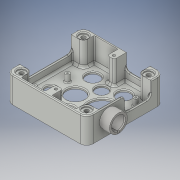
# Autodesk Inventor part: NUCBasePCB
Saved by Autodesk Inventor 2016 (Build 200138000, 138)
## iProperties
Created: 2015-09-23
Part Number: NUCBasePCB
Material: Generic
Document SubType Name: Modeling
Designer: lachesis
Density: 1 g/cm^3
Appearance: Default
Author: lachesis
Autodesk Inventor part; units mm, degrees
ref_plane "YZ Plane" through (0, 0, 0) normal (1, 0, 0) x (0, 1, 0)
ref_plane "XZ Plane" through (0, 0, 0) normal (0, 1, 0) x (-1, 0, 0)
ref_plane "XY Plane" through (0, 0, 0) normal (0, 0, 1) x (1, 0, 0)
sketch "Sketch1" plane through (0, 0, 0) normal (0, 1, 0) x (-1, 0, 0)
  line L0 (58.42, 56.134) -> (-58.42, 56.134)
  line L1 (-58.42, 56.134) -> (-58.42, -56.134)
  line L2 (-58.42, -56.134) -> (58.42, -56.134)
  line L3 (58.42, -56.134) -> (58.42, 56.134)
  point P0 (0, 0)
  point P1 (0, -56.134)
  point P2 (58.42, 0)
  dimension "d0" = 112.268
  dimension "d1" = 116.84
  constraints: 8 end point, 2 midpoint, 2 parallel, 1 horizontal, 1 horizontal alignment, 1 perpendicular, 1 vertical alignment
  measures "d0" distance of L2.end L0.start
  measures "d1" distance of L1.end L2.end
extrude "Extrusion1" add sketch "Sketch1" along normal blind 37.335
sketch "Sketch2" plane through (0, 37.335, 0) normal (0, 1, 0) x (1, 0, 0)
  line L0 (58.42, -56.134) -> (58.42, 56.134) projected
  line L1 (58.42, 56.134) -> (-58.42, 56.134) projected
  line L2 (-58.42, -56.134) -> (58.42, -56.134) projected
  line L3 (-58.42, 56.134) -> (-58.42, -56.134) projected
  point P0 (0, 0)
  point P1 (47.244, 44.958)
  point P2 (47.244, -44.958)
  point P3 (-47.244, 44.958)
  point P4 (-47.244, -44.958)
  dimension "d4" = 11.176
  dimension "d5" = 11.176
  dimension "d6" = 11.176
  dimension "d7" = 11.176
  constraints: 2 horizontal alignment, 2 vertical alignment
  measures "d4" distance from line of L0 point (47.244, 44.958)
  measures "d5" distance from line of L1 point (47.244, 44.958)
  measures "d6" distance from line of L2 point (-47.244, -44.958)
  measures "d7" distance from line of L3 point (-47.244, -44.958)
hole "Hole1" at (47.244, 37.335, -44.958) at (47.244, 37.335, 44.958) at (-47.244, 37.335, -44.958) at (-47.244, 37.335, 44.958) direction (0, -1, 0) diameter 3.302 end through all counterbore diameter 5.969 counterbore depth 31.75
sketch "Sketch3" plane through (0, 37.335, 0) normal (0, 1, 0) x (1, 0, 0)
  circle A0 centre (47.244, 44.958) radius 2.9845 projected
  circle A1 centre (47.244, -44.958) radius 2.9845 projected
  circle A2 centre (-47.244, 44.958) radius 2.9845 projected
  circle A3 centre (-47.244, -44.958) radius 2.9845 projected
  circle A4 centre (47.244, 44.958) radius 1.651 projected
  circle A5 centre (47.244, -44.958) radius 1.651 projected
  circle A6 centre (-47.244, -44.958) radius 1.651 projected
  point P0 (0, 0)
  constraints: 4 coincident
hole "Hole2" at (47.244, 37.335, -44.958) at (47.244, 37.335, 44.958) at (-47.244, 37.335, 44.958) at (-47.244, 37.335, -44.958) direction (0, -1, 0) diameter 12.065 depth 2.413
sketch "Sketch5" plane through (0, 0, 0) normal (0, -1, 0) x (1, 0, 0)
  circle A0 centre (-47.244, 44.958) radius 1.651 projected
  circle A1 centre (-47.244, -44.958) radius 1.651 projected
  point P0 (0, 0)
  point P1 (0, 42.164)
  point P2 (0, -42.164)
  dimension "d25" = 47.244
  dimension "d26" = 2.794
  dimension "d27" = 2.794
  constraints: 1 vertical alignment
  measures "d25" horizontal distance of A0.centre point (0, 42.164)
  measures "d26" vertical distance of A0.centre point (0, 42.164)
  measures "d27" vertical distance of A1.centre point (0, -42.164)
hole "Hole3" at (0, 0, 42.164) at (0, 0, -42.164) direction (0, 1, 0) diameter 3.9116 end through all counterbore diameter 6.604 counterbore depth 25.146
sketch "Sketch6" plane through (0, 37.335, 0) normal (0, 1, 0) x (1, 0, 0)
  circle A0 centre (0, -42.164) radius 1.9558 projected
  circle A1 centre (0, 42.164) radius 1.9558 projected
  circle A2 centre (-47.244, -44.958) radius 6.0325 projected
  circle A3 centre (47.244, 44.958) radius 6.0325 projected
  circle A4 centre (47.244, -44.958) radius 6.0325 projected
  circle A5 centre (-47.244, 44.958) radius 6.0325 projected
  line L0 (-58.42, -56.134) -> (58.42, -56.134) projected
  line L1 (58.42, -56.134) -> (58.42, 56.134) projected
  line L2 (58.42, 56.134) -> (-58.42, 56.134) projected
  line L3 (-58.42, 56.134) -> (-58.42, -56.134) projected
  line L4 (39.624, 52.959) -> (39.624, 37.338)
  line L5 (39.624, 37.338) -> (55.245, 37.338)
  line L6 (55.245, 37.338) -> (55.245, -37.338)
  line L7 (55.245, -37.338) -> (39.624, -37.338)
  line L8 (39.624, -37.338) -> (39.624, -52.959)
  line L9 (-39.624, -52.959) -> (-39.624, -37.338)
  line L10 (-39.624, -37.338) -> (-55.245, -37.338)
  line L11 (-55.245, -37.338) -> (-55.245, 37.338)
  line L12 (-55.245, 37.338) -> (-39.624, 37.338)
  line L13 (-39.624, 37.338) -> (-39.624, 52.959)
  line L14 (-39.624, -52.959) -> (-5.08, -52.959)
  line L15 (-5.08, -52.959) -> (-5.08, -37.338)
  line L16 (-5.08, -37.338) -> (5.08, -37.338)
  line L17 (5.08, -37.338) -> (5.08, -52.959)
  line L18 (5.08, -52.959) -> (39.624, -52.959)
  line L19 (-39.624, 52.959) -> (-5.08, 52.959)
  line L20 (-5.08, 52.959) -> (-5.08, 37.338)
  line L21 (-5.08, 37.338) -> (5.08, 37.338)
  line L22 (5.08, 37.338) -> (5.08, 52.959)
  line L23 (5.08, 52.959) -> (39.624, 52.959)
  point P0 (0, 0)
  dimension "d36" = 3.175
  dimension "d37" = 15.621
  dimension "d38" = 15.621
  dimension "d39" = 15.621
  dimension "d41" = 3.175
  dimension "d42" = 5.08
  dimension "d43" = 5.08
  dimension "d44" = 3.175
  dimension "d45" = 3.175
  constraints: 40 end point, 15 perpendicular, 7 equal length, 3 point on line, 2 horizontal, 1 collinear, 1 vertical
  measures "d36" distance between parallel lines of L3 L11
  measures "d37" distance of L12.end L13.end
  measures "d38" distance of L7.end L8.end
  measures "d39" distance of L9.end L10.end
  measures "d41" distance between parallel lines of L1 L6
  measures "d42" distance from line of A0.centre L17
  measures "d43" distance from line of A0.centre L15
  measures "d44" distance between parallel lines of L0 L14
  measures "d45" distance between parallel lines of L2 L19
extrude "Extrusion2" cut sketch "Sketch6" against normal blind 34.16 contours L4 L5 L6 L7 L8 L18 L17 L16 L15 L14 L9 L10 L11 L12 L13 L19 L20 L21 L22 L23
sketch "Sketch8" plane through (0, 3.175, 0) normal (0, 1, 0) x (1, 0, 0)
  line L0 (-50.8, 35.56) -> (50.8, 35.56)
  line L1 (50.8, 35.56) -> (50.8, -35.56)
  line L2 (50.8, -35.56) -> (-50.8, -35.56)
  line L3 (-50.8, -35.56) -> (-50.8, 35.56)
  line L4 (-55.245, 37.338) -> (-39.624, 37.338) projected
  line L5 (-55.245, -37.338) -> (-55.245, 37.338) projected
  line L6 (55.245, 37.338) -> (55.245, -37.338) projected
  line L7 (55.245, -37.338) -> (39.624, -37.338) projected
  line L8 (0, 35.56) -> (0, -35.56)
  circle A0 centre (-35.56, 10.16) radius 3.175
  circle A1 centre (44.45, 29.21) radius 3.175
  circle A2 centre (-44.45, -29.21) radius 3.175
  circle A3 centre (44.45, -29.21) radius 3.175
  point P0 (0, 0)
  point P1 (0, 0)
  dimension "d51" = 101.6
  dimension "d52" = 71.12
  dimension "d53" = 6.35
  dimension "d54" = 6.35
  dimension "d55" = 6.35
  dimension "d56" = 6.35
  dimension "d57" = 6.35
  dimension "d58" = 45.72
  dimension "d59" = 15.24
  constraints: 10 end point, 4 centre point, 3 equal radius, 3 midpoint, 2 parallel, 1 coincident, 1 horizontal, 1 horizontal alignment, 1 perpendicular, 1 vertical alignment
  measures "d51" distance of L0.start L0.end
  measures "d52" distance of L2.end L0.start
  measures "d53" distance from line of L0 A1.centre
  measures "d54" distance from line of A1.centre L1
  measures "d55" distance from line of L2 A2.centre
  measures "d56" diameter of A0
  measures "d57" distance from line of L3 A2.centre
  measures "d58" vertical distance of L2.end A0.centre
  measures "d59" horizontal distance of L2.end A0.centre
extrude "Extrusion4" add sketch "Sketch8" along normal blind 10.16 contours A0 | A1 | A2 | A3
sketch "Sketch9" plane through (-35.56, 13.335, -10.16) normal (0, 1, 0) x (1, 0, 0)
  circle A0 centre (-8.89, -39.37) radius 3.175 projected
  circle A1 centre (80.01, -39.37) radius 3.175 projected
  circle A2 centre (80.01, 19.05) radius 3.175 projected
  circle A3 centre (0, 0) radius 3.175 projected
  circle A4 centre (-8.89, -39.37) radius 3.175 projected
  point P0 (35.56, -10.16)
  constraints: 4 coincident
hole "Hole4" at (-35.56, 13.335, -10.16) at (-44.45, 13.335, 29.21) at (44.45, 13.335, -29.21) at (44.45, 13.335, 29.21) direction (0, -1, 0) diameter 2.2606 depth 10.16
sketch "Sketch10" plane through (-58.42, 0, -56.134) normal (-1, 0, 0) x (0, 0, 1)
  line L0 (93.472, 37.335) -> (93.472, 3.175) projected
  line L1 (18.796, 37.335) -> (18.796, 3.175) projected
  line L2 (93.472, 3.175) -> (18.796, 3.175) projected
  line L3 (93.472, 37.335) -> (18.796, 37.335) projected
  line L4 (18.796, 37.335) -> (18.796, 3.175) projected
  line L5 (93.472, 37.335) -> (93.472, 3.175) projected
  line L6 (18.796, 37.335) -> (93.472, 37.335)
  line L7 (93.472, 37.335) -> (93.472, 15.3416)
  line L8 (93.472, 15.3416) -> (18.796, 15.3416)
  line L9 (18.796, 15.3416) -> (18.796, 37.335)
  point P0 (56.134, 0)
  dimension "d69" = 12.1666
  constraints: 8 end point, 2 parallel, 1 horizontal, 1 perpendicular, 1 point on line
  measures "d69" distance between parallel lines of L2 L8
extrude "Extrusion5" cut sketch "Sketch10" against normal up to surface (3.175 mm away) contours L0 L8 L1 L3
sketch "Sketch11" plane through (58.42, 0, 56.134) normal (1, 0, 0) x (0, 0, -1)
  line L0 (93.472, 37.335) -> (93.472, 3.175) projected
  line L1 (18.796, 37.335) -> (18.796, 3.175) projected
  line L2 (93.472, 37.335) -> (18.796, 37.335) projected
  line L3 (93.472, 15.3416) -> (18.796, 15.3416) projected
  line L4 (18.796, 37.335) -> (93.472, 37.335)
  line L5 (93.472, 37.335) -> (93.472, 15.3416)
  line L6 (93.472, 15.3416) -> (18.796, 15.3416)
  line L7 (18.796, 15.3416) -> (18.796, 37.335)
  line L8 (0, 37.335) -> (112.268, 37.335) projected
  line L9 (56.134, 37.335) -> (56.134, 15.3416)
  point P0 (56.134, 0)
  constraints: 10 end point, 2 midpoint, 2 parallel, 1 horizontal, 1 perpendicular
extrude "Extrusion6" cut sketch "Sketch11" against normal up to surface (3.175 mm away) contours L0 L3 L9 L2
sketch "Sketch12" plane through (58.42, 0, -56.134) normal (0, 0, -1) x (-1, 0, 0)
  line L0 (53.34, 37.335) -> (18.796, 37.335) projected
  line L1 (53.34, 37.335) -> (53.34, 3.175) projected
  line L2 (53.34, 3.175) -> (18.796, 3.175) projected
  line L3 (18.796, 37.335) -> (18.796, 3.175) projected
  line L4 (98.044, 37.335) -> (63.5, 37.335) projected
  line L5 (98.044, 37.335) -> (98.044, 3.175) projected
  line L6 (98.044, 3.175) -> (63.5, 3.175) projected
  line L7 (63.5, 37.335) -> (63.5, 3.175) projected
  line L8 (18.796, 37.335) -> (53.34, 37.335)
  line L9 (53.34, 37.335) -> (53.34, 15.3416)
  line L10 (53.34, 15.3416) -> (18.796, 15.3416)
  line L11 (18.796, 15.3416) -> (18.796, 37.335)
  point P0 (58.42, 0)
  dimension "d74" = 12.1666
  constraints: 8 end point, 2 parallel, 1 horizontal, 1 perpendicular, 1 point on line
  measures "d74" distance between parallel lines of L2 L10
extrude "Extrusion7" cut sketch "Sketch12" against normal up to surface (3.175 mm away) contours L1 L10 L3 L0
fillet "Fillet1" radius 9.525 4 edges at (58.42, 18.6675, 56.134) (58.42, 18.6675, -56.134) (-58.42, 18.6675, 56.134) (-58.42, 18.6675, -56.134)
fillet "Fillet2" radius 6.35 7 edges at (-56.8325, 15.3416, 37.338) (56.8325, 15.3416, 0) (56.8325, 37.335, 0) (39.624, 15.3416, -54.5465) (-56.8325, 15.3416, -37.338) (5.08, 15.3416, -54.5465) (56.8325, 15.3416, -37.338)
fillet "Fillet3" radius 6.35 4 edges at (-39.624, 20.255, -37.338) (39.624, 20.255, -37.338) (39.624, 20.255, 37.338) (-39.624, 20.255, 37.338)
fillet "Fillet4" radius 3.175 4 edges at (-5.08, 20.255, 37.338) (5.08, 20.255, 37.338) (-5.08, 20.255, -37.338) (5.08, 20.255, -37.338)
fillet "Fillet5" radius 1.27 39 edges at (-58.42, 17.2015, -35.4781) (-58.42, 29.5133, -37.338) (-58.42, 17.2015, 35.4781) (-58.42, 29.5133, 37.338) (-58.42, 15.3416, 0) (-55.245, 17.2015, 35.4781) (-55.245, 17.2015, -35.4781) (-55.245, 15.3416, 0) (55.245, 17.2015, -35.4781) (55.245, 17.2015, -1.8599) (55.245, 26.3383, 0) (55.245, 35.4751, 1.8599) (55.245, 37.335, 21.844) (55.245, 15.3416, -18.669) (58.42, 17.2015, -1.8599) (58.42, 26.3383, 0) (58.42, 35.4751, 1.8599) (58.42, 37.335, 26.4795) (55.6302, 37.335, 53.3442) (0, 37.335, 56.134) (-55.6302, 37.335, 53.3442) (-58.42, 37.335, 41.9735) (58.42, 17.2015, -35.4781) (58.42, 29.5133, -37.338) (58.42, 15.3416, -18.669) (37.7641, 17.2015, -56.134) (39.624, 29.5133, -56.134) (6.9399, 17.2015, -56.134) (5.08, 29.5133, -56.134) (22.352, 15.3416, -56.134) (6.9399, 17.2015, -52.959) (37.7641, 17.2015, -52.959) (22.352, 15.3416, -52.959) (-55.6302, 37.335, -53.3442) (-21.9075, 37.335, -56.134) (-58.42, 37.335, -41.9735) (55.6302, 37.335, -53.3442) (58.42, 37.335, -41.9735) (44.2595, 37.335, -56.134)
fillet "Fillet6" radius 3.175 28 edges at (55.245, 3.175, 0) (-22.352, 3.175, 52.959) (-4.1501, 3.175, 38.2679) (0, 3.175, 37.338) (4.1501, 3.175, 38.2679) (5.08, 3.175, 46.736) (-5.08, 3.175, 46.736) (22.352, 3.175, 52.959) (41.4839, 3.175, 39.1979) (50.6095, 3.175, 37.338) (39.624, 3.175, 48.3235) (-55.245, 3.175, 0) (-39.624, 3.175, -48.3235) (-50.6095, 3.175, -37.338) (-41.4839, 3.175, -39.1979) (-22.352, 3.175, -52.959) (4.1501, 3.175, -38.2679) (0, 3.175, -37.338) (-4.1501, 3.175, -38.2679) (-5.08, 3.175, -46.736) (5.08, 3.175, -46.736) (22.352, 3.175, -52.959) (50.6095, 3.175, -37.338) (39.624, 3.175, -48.3235) (41.4839, 3.175, -39.1979) (-41.4839, 3.175, 39.1979) (-50.6095, 3.175, 37.338) (-39.624, 3.175, 48.3235)
fillet "Fillet7" radius 1.27 4 edges at (-47.625, 3.175, 29.21) (41.275, 3.175, 29.21) (41.275, 3.175, -29.21) (-38.735, 3.175, -10.16)
fillet "Fillet8" radius 1.27 4 edges at (47.244, 37.335, -50.9905) (-47.244, 37.335, -50.9905) (-47.244, 37.335, 38.9255) (47.244, 37.335, 38.9255)
fillet "Fillet9" radius 1.27 30 edges at (-38.6941, 4.1049, -52.0291) (-39.624, 21.8425, -52.959) (-54.3151, 4.1049, -36.4081) (-55.6648, 19.629, -37.338) (-55.245, 11.9147, -37.338) (6.0099, 4.1049, -52.0291) (5.08, 19.5076, -53.3379) (5.08, 11.9147, -52.959) (38.6941, 4.1049, 52.0291) (39.624, 21.8425, 52.959) (54.3151, 4.1049, 36.4081) (55.617, 36.963, 37.338) (55.245, 21.2075, 37.338) (-6.0099, 4.1049, 52.0291) (-5.08, 21.8425, 52.959) (6.0099, 4.1049, 52.0291) (5.08, 21.8425, 52.959) (-38.6941, 4.1049, 52.0291) (-39.624, 21.8425, 52.959) (-54.3151, 4.1049, 36.4081) (-55.6648, 19.629, 37.338) (-55.245, 11.9147, 37.338) (-6.0099, 4.1049, -52.0291) (-5.08, 21.8425, -52.959) (38.6941, 4.1049, -52.0291) (39.624, 19.629, -53.3788) (39.624, 11.9147, -52.959) (54.3151, 4.1049, -36.4081) (55.6648, 19.629, -37.338) (55.245, 11.9147, -37.338)
sketch "Sketch13" plane through (0, 3.175, 0) normal (0, 1, 0) x (1, 0, 0)
  line L0 (-27.7495, -41.0845) -> (-16.9545, -41.0845) construction
  line L1 (-27.7495, -46.609) -> (-16.9545, -46.609)
  line L2 (-16.9545, -35.56) -> (-27.7495, -35.56)
  arc A0 (-27.7495, -35.56) -> (-27.7495, -46.609) centre (-27.7495, -41.0845) ccw
  arc A1 (-16.9545, -46.609) -> (-16.9545, -35.56) centre (-16.9545, -41.0845) ccw
  line L3 (16.9545, -41.0845) -> (27.7495, -41.0845) construction
  line L4 (16.9545, -35.56) -> (27.7495, -35.56)
  line L5 (27.7495, -46.609) -> (16.9545, -46.609)
  arc A2 (16.9545, -35.56) -> (16.9545, -46.609) centre (16.9545, -41.0845) ccw
  arc A3 (27.7495, -46.609) -> (27.7495, -35.56) centre (27.7495, -41.0845) ccw
  line L6 (-6.35, -52.959) -> (-38.354, -52.959) projected
  line L7 (-38.354, -52.959) -> (-6.35, -52.959) projected
  line L8 (38.354, -52.959) -> (6.35, -52.959) projected
  line L9 (6.35, -52.959) -> (38.354, -52.959) projected
  line L10 (-6.35, -52.959) -> (-38.354, -52.959) projected
  line L11 (38.354, -52.959) -> (6.35, -52.959) projected
  line L12 (-38.354, -52.959) -> (-6.35, -52.959) projected
  line L13 (-8.255, -49.784) -> (-36.449, -49.784) projected
  line L14 (36.449, -49.784) -> (8.255, -49.784) projected
  line L15 (-36.449, -49.784) -> (-36.449, -43.688) projected
  line L16 (-8.255, -40.513) -> (-8.255, -49.784) projected
  circle A4 centre (44.45, 29.21) radius 4.445 projected
  circle A5 centre (-44.45, -29.21) radius 4.445 projected
  line L17 (-52.07, 34.163) -> (-45.974, 34.163) projected
  line L18 (-52.07, -34.163) -> (-52.07, 34.163) projected
  line L19 (-45.974, -34.163) -> (-52.07, -34.163) projected
  arc A6 (-36.449, -43.688) -> (-45.974, -34.163) centre (-45.974, -43.688) ccw projected
  line L20 (-36.449, -49.784) -> (-36.449, -43.688) projected
  line L21 (-8.255, -49.784) -> (-36.449, -49.784) projected
  line L22 (-8.255, -40.513) -> (-8.255, -49.784) projected
  arc A7 (-1.905, -34.163) -> (-8.255, -40.513) centre (-1.905, -40.513) ccw projected
  line L23 (1.905, -34.163) -> (-1.905, -34.163) projected
  arc A8 (8.255, -40.513) -> (1.905, -34.163) centre (1.905, -40.513) ccw projected
  line L24 (8.255, -49.784) -> (8.255, -40.513) projected
  line L25 (36.449, -49.784) -> (8.255, -49.784) projected
  line L26 (36.449, -43.688) -> (36.449, -49.784) projected
  arc A9 (45.974, -34.163) -> (36.449, -43.688) centre (45.974, -43.688) ccw projected
  line L27 (52.07, -34.163) -> (45.974, -34.163) projected
  line L28 (52.07, 34.163) -> (52.07, -34.163) projected
  line L29 (45.974, 34.163) -> (52.07, 34.163) projected
  arc A10 (36.449, 43.688) -> (45.974, 34.163) centre (45.974, 43.688) ccw projected
  line L30 (36.449, 49.784) -> (36.449, 43.688) projected
  line L31 (8.255, 49.784) -> (36.449, 49.784) projected
  line L32 (8.255, 40.513) -> (8.255, 49.784) projected
  arc A11 (1.905, 34.163) -> (8.255, 40.513) centre (1.905, 40.513) ccw projected
  line L33 (-1.905, 34.163) -> (1.905, 34.163) projected
  arc A12 (-8.255, 40.513) -> (-1.905, 34.163) centre (-1.905, 40.513) ccw projected
  line L34 (-8.255, 49.784) -> (-8.255, 40.513) projected
  line L35 (-36.449, 49.784) -> (-8.255, 49.784) projected
  line L36 (-36.449, 43.688) -> (-36.449, 49.784) projected
  arc A13 (-45.974, 34.163) -> (-36.449, 43.688) centre (-45.974, 43.688) ccw projected
  circle A14 centre (44.45, -29.21) radius 4.445 projected
  circle A15 centre (-35.56, 10.16) radius 4.445 projected
  point P0 (0, 0)
  point P1 (-22.352, -41.0845)
  point P2 (22.352, -41.0845)
  dimension "d86" = 3.175
  dimension "d87" = 3.175
  dimension "d88" = 3.175
  dimension "d89" = 3.175
  dimension "d90" = 11.049
  constraints: 16 end point, 8 point on circle, 8 tangent, 4 centre point, 3 parallel, 2 midpoint, 2 point on line, 1 equal radius, 1 horizontal
  measures "d86" distance between parallel lines of L1 L13
  measures "d87" distance edge to line of A1 L22
  measures "d88" distance edge to line of A0 L15
  measures "d89" distance edge to line of A2 L24
  measures "d90" distance between parallel lines of L1 L2
extrude "Extrusion8" cut sketch "Sketch13" against normal through all contours A0 L2 A1 L1 | L4 A3 L5 A2
fillet "Fillet10" radius 1.27 8 edges at (-33.274, 3.175, 41.0845) (-22.352, 3.175, 35.56) (-11.43, 3.175, 41.0845) (-22.352, 3.175, 46.609) (11.43, 3.175, 41.0845) (22.352, 3.175, 35.56) (33.274, 3.175, 41.0845) (22.352, 3.175, 46.609)
sketch "Sketch14" plane through (0, 0, 0) normal (0, -1, 0) x (1, 0, 0)
  arc A0 (-16.9545, 35.56) -> (-16.9545, 46.609) centre (-16.9545, 41.0845) ccw projected
  line L0 (-16.9545, 35.56) -> (-27.7495, 35.56) projected
  arc A1 (-27.7495, 46.609) -> (-27.7495, 35.56) centre (-27.7495, 41.0845) ccw projected
  line L1 (-27.7495, 46.609) -> (-16.9545, 46.609) projected
  arc A2 (16.9545, 46.609) -> (16.9545, 35.56) centre (16.9545, 41.0845) ccw projected
  line L2 (16.9545, 46.609) -> (27.7495, 46.609) projected
  arc A3 (27.7495, 35.56) -> (27.7495, 46.609) centre (27.7495, 41.0845) ccw projected
  line L3 (27.7495, 35.56) -> (16.9545, 35.56) projected
  arc A4 (-58.42, -46.609) -> (-48.895, -56.134) centre (-48.895, -46.609) ccw projected
  line L4 (48.895, -56.134) -> (-48.895, -56.134) projected
  arc A5 (48.895, -56.134) -> (58.42, -46.609) centre (48.895, -46.609) ccw projected
  line L5 (58.42, 46.609) -> (58.42, -46.609) projected
  arc A6 (58.42, 46.609) -> (48.895, 56.134) centre (48.895, 46.609) ccw projected
  line L6 (-48.895, 56.134) -> (48.895, 56.134) projected
  arc A7 (-48.895, 56.134) -> (-58.42, 46.609) centre (-48.895, 46.609) ccw projected
  line L7 (-58.42, -46.609) -> (-58.42, 46.609) projected
  circle A8 centre (-47.244, 44.958) radius 1.651 projected
  circle A9 centre (47.244, 44.958) radius 1.651 projected
  circle A10 centre (47.244, -44.958) radius 1.651 projected
  circle A11 centre (-47.244, -44.958) radius 1.651 projected
  circle A12 centre (0, -42.164) radius 3.302 projected
  circle A13 centre (0, 42.164) radius 3.302 projected
  circle A14 centre (0, -24.0273) radius 8.4847
  circle A15 centre (0, 24.0273) radius 8.4847
  circle A16 centre (-14.0463, 0) radius 12.9972
  circle A17 centre (25.5105, 0) radius 20.2095
  line L8 (-52.07, 34.163) -> (-52.07, -34.163) projected
  line L9 (52.07, -34.163) -> (52.07, 34.163) projected
  circle A18 centre (0, -42.164) radius 1.9558 construction
  circle A19 centre (0, 42.164) radius 3.302 construction
  line L10 (0, -42.164) -> (0, 42.164) construction
  line L11 (-1.905, 37.338) -> (1.905, 37.338) construction
  line L12 (58.42, 46.609) -> (58.42, -46.609) construction
  line L13 (58.42, 0) -> (-58.42, 0) construction
  arc A20 (-36.449, -43.688) -> (-45.974, -34.163) centre (-45.974, -43.688) ccw projected
  arc A21 (45.974, -34.163) -> (36.449, -43.688) centre (45.974, -43.688) ccw projected
  line L14 (-22.9869, -36.3219) -> (-22.9869, -37.0473) construction
  line L15 (8.255, -49.784) -> (36.449, -49.784) projected
  line L16 (-36.449, -49.784) -> (-8.255, -49.784) projected
  circle A22 centre (22.4512, -33.7877) radius 9.6463
  circle A23 centre (-22.4512, -33.7877) radius 9.6463
  circle A24 centre (-35.56, -10.16) radius 4.445 projected
  circle A25 centre (-38.1543, 11.9624) radius 7.5657
  circle A26 centre (-44.45, 29.21) radius 4.445 projected
  point P0 (0, 0)
  dimension "d95" = 6.35
  dimension "d96" = 6.35
  dimension "d97" = 6.35
  dimension "d98" = 6.35
  dimension "d99" = 6.35
  dimension "d101" = 6.35
  dimension "d104" = 6.35
  dimension "d127" = 6.35
  dimension "d128" = 6.35
  dimension "d130" = 6.35
  dimension "d131" = 6.35
  dimension "d135" = 6.35
  dimension "d136" = 6.35
  dimension "d137" = 6.35
  dimension "d138" = 6.35
  dimension "d139" = 6.35
  dimension "d141" = 6.35
  constraints: 8 end point, 7 centre point, 4 point on line, 2 midpoint, 1 perpendicular
  measures "d101" distance edge to line of A17 L9
  measures "d127" distance edge to line of A22 L15
  measures "d131" distance edge to line of A23 L16
  measures "d139" distance edge to line of A25 L8
extrude "Extrusion10" cut sketch "Sketch14" against normal up to surface (3.175 mm away) contours A14 | A15 | A16 | A17 | A22 | A23 | A25
fillet "Fillet12" radius 1.27 7 edges at (-32.0975, 3.175, -33.7877) (-27.0434, 3.175, 0) (-45.72, 3.175, 11.9624) (-8.4847, 3.175, -24.0273) (12.8048, 3.175, -33.7877) (5.3009, 3.175, 0) (-8.4847, 3.175, 24.0273)
sketch "Sketch22" plane through (58.42, 0, 46.609) normal (1, 0, 0) x (0, 0, -1)
  circle A0 centre (22.2555, 21.8425) radius 13
  line L0 (0, 36.065) -> (40.259, 36.065) projected
  line L1 (10.541, 6.35) -> (82.677, 6.35) projected
  line L2 (9.271, 6.35) -> (9.271, 36.065) projected
  line L3 (9.271, 37.335) -> (9.271, 6.35) projected
  point P0 (46.609, 0)
  point P1 (9.271, 21.2075)
  point P2 (9.271, 21.8425)
  dimension "d166" = 26
  constraints: 2 midpoint, 1 coincident, 1 horizontal alignment, 3 other
extrude "Extrusion17" add sketch "Sketch22" along normal blind 14.5
sketch "Sketch21" plane through (55.245, 21.6916, 1.27) normal (-1, 0, 0) x (0, 0, 1)
  circle A0 centre (23.0835, 0.1509) radius 11.5
  circle A1 centre (23.0835, 0.1509) radius 13 projected
  point P0 (-1.27, -21.6916)
  dimension "d162" = 23
  constraints: 1 centre point, 1 coincident
  measures "d162" diameter of A0
extrude "Extrusion16" cut sketch "Sketch21" against normal blind 15.675 contours A0
sketch "Sketch23" plane through (72.92, 21.8425, 24.3535) normal (1, 0, 0) x (0, 0, -1)
  circle A0 centre (0, 0) radius 13 projected
  circle A1 centre (0, 0) radius 11.5 projected
  circle A2 centre (0, 0) radius 10.1
  point P0 (24.3535, -21.8425)
  dimension "d170" = 20.2
  constraints: 1 centre point, 1 coincident
  measures "d170" diameter of A2
extrude "Extrusion18" cut sketch "Sketch23" against normal blind 14.5 contours A2
sketch "Sketch24" plane through (72.92, 21.8425, 24.3535) normal (1, 0, 0) x (0, 0, -1)
  circle A0 centre (0, 0) radius 10.1 projected
  circle A1 centre (0, 0) radius 13 projected
  circle A2 centre (0, 0) radius 10.1 projected
  line L0 (-1.1, -10.0399) -> (-1.1, -12.2399)
  line L1 (-1.1, -12.2399) -> (1.1, -12.2399)
  line L2 (1.1, -12.2399) -> (1.1, -10.0399)
  point P0 (24.3535, -21.8425)
  dimension "d173" = 2.2
  dimension "d174" = 2.2
  constraints: 6 end point, 4 point on circle, 2 perpendicular, 1 horizontal, 1 parallel
  measures "d173" distance of L0.start L0.end
  measures "d174" distance of L0.end L1.end
extrude "Extrusion19" cut sketch "Sketch24" against normal up to next contours A0 L2 L1 L0
equation "\"d5\" = d4"
equation "\"d6\" = d4"
equation "\"d7\" = d4"
equation "\"d38\" = d37"
equation "\"d39\" = d37"
equation "\"d41\" = d36"
equation "\"d43\" = d42"
equation "\"d44\" = d36"
equation "\"d45\" = d36"
equation "\"d54\" = d53"
equation "\"d55\" = d54"
equation "\"d57\" = d54"
equation "\"d89\" = d88"
body "Solid1"
